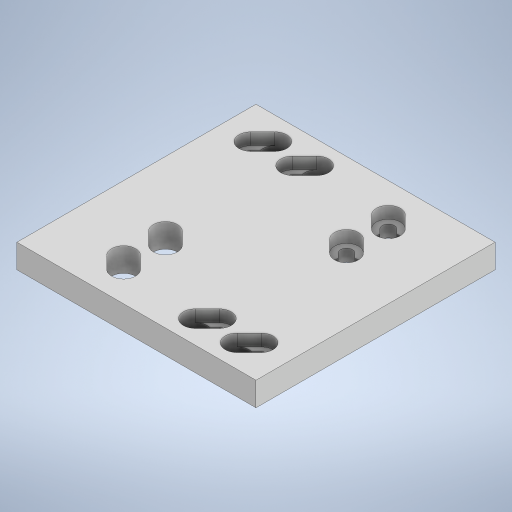
# Autodesk Inventor part: middle
Saved by Autodesk Inventor 2023 (Build 270158000, 158)
## iProperties
Created: 2023-08-09
Part Number: middle
Material: Generic
Document SubType Name: Modeling
Designer: AxLab
Density: 1 g/cm^3
Appearance: Default
Author: AxLab
Autodesk Inventor part; units mm, degrees
ref_plane "YZ Plane" through (0, 0, 0) normal (1, 0, 0) x (0, 1, 0)
ref_plane "XZ Plane" through (0, 0, 0) normal (0, 1, 0) x (-1, 0, 0)
ref_plane "XY Plane" through (0, 0, 0) normal (0, 0, 1) x (1, 0, 0)
sketch "Sketch6" plane through (0, 0, 0) normal (0, 1, 0) x (-1, 0, 0)
  line L0 (20, 20) -> (-20, 20)
  line L1 (-20, 20) -> (-20, -20)
  line L2 (-20, -20) -> (20, -20)
  line L3 (20, -20) -> (20, 20)
  line L4 (20, 20) -> (-20, -20) construction
  line L5 (-20, 20) -> (20, -20) construction
  line L6 (2.15, 11.15) -> (-2.15, 11.15)
  line L7 (-2.15, 11.15) -> (-2.15, -11.15)
  line L8 (-2.15, -11.15) -> (2.15, -11.15)
  line L9 (2.15, -11.15) -> (2.15, 11.15)
  line L10 (2.15, 11.15) -> (-2.15, -11.15) construction
  line L11 (-2.15, 11.15) -> (2.15, -11.15) construction
  line L12 (2.15, -11.15) -> (-20, -11.15)
  line L13 (-20, -11.15) -> (-20, -20)
  line L14 (-20, -20) -> (2.15, -20)
  line L15 (2.15, -20) -> (2.15, -11.15)
  line L16 (-2.15, 11.15) -> (20, 11.15)
  line L17 (20, 11.15) -> (20, 20)
  line L18 (20, 20) -> (-2.15, 20)
  line L19 (-2.15, 20) -> (-2.15, 11.15)
  line L20 (-20, -11.15) -> (-15, -11.15)
  line L21 (-15, -11.15) -> (-15, -14.15)
  line L22 (-15, -14.15) -> (-20, -14.15)
  line L23 (-20, -14.15) -> (-20, -11.15)
  line L24 (-20, -11.15) -> (-8, -11.15)
  line L25 (-8, -11.15) -> (-8, -14.15)
  line L26 (-8, -14.15) -> (-20, -14.15)
  line L27 (-20, -14.15) -> (-20, -11.15)
  line L28 (-2.15, 20) -> (-7.15, 20)
  line L29 (-7.15, 20) -> (-7.15, 15)
  line L30 (-7.15, 15) -> (-2.15, 15)
  line L31 (-2.15, 15) -> (-2.15, 20)
  line L32 (-2.15, 20) -> (-7.15, 20)
  line L33 (-7.15, 20) -> (-7.15, 8)
  line L34 (-7.15, 8) -> (-2.15, 8)
  line L35 (-2.15, 8) -> (-2.15, 20)
  line L36 (20, 11.15) -> (15, 11.15)
  line L37 (15, 11.15) -> (15, 14.15)
  line L38 (15, 14.15) -> (20, 14.15)
  line L39 (20, 14.15) -> (20, 11.15)
  line L40 (20, 11.15) -> (8, 11.15)
  line L41 (8, 11.15) -> (8, 14.15)
  line L42 (8, 14.15) -> (20, 14.15)
  line L43 (20, 14.15) -> (20, 11.15)
  line L44 (2.15, -20) -> (7.15, -20)
  line L45 (7.15, -20) -> (7.15, -15)
  line L46 (7.15, -15) -> (2.15, -15)
  line L47 (2.15, -15) -> (2.15, -20)
  line L48 (2.15, -20) -> (7.15, -20)
  line L49 (7.15, -20) -> (7.15, -8)
  line L50 (7.15, -8) -> (2.15, -8)
  line L51 (2.15, -8) -> (2.15, -20)
  circle A0 centre (-13, -16.15) radius 2
  circle A1 centre (-6, -16.15) radius 2
  circle A2 centre (9.15, -13) radius 2
  circle A3 centre (9.15, -6) radius 2
  circle A4 centre (6, 16.15) radius 2
  circle A5 centre (13, 16.15) radius 2
  circle A6 centre (-9.15, 6) radius 2
  circle A7 centre (-9.15, 13) radius 2
  line L52 (-13, -16.15) -> (-15, -16.15)
  line L53 (-15, -16.15) -> (-15, -14.15)
  line L54 (-15, -14.15) -> (-13, -14.15)
  line L55 (-13, -14.15) -> (-13, -16.15)
  line L56 (-6, -16.15) -> (-8, -16.15)
  line L57 (-8, -16.15) -> (-8, -14.15)
  line L58 (-8, -14.15) -> (-6, -14.15)
  line L59 (-6, -14.15) -> (-6, -16.15)
  line L60 (9.15, -13) -> (7.15, -13)
  line L61 (7.15, -13) -> (7.15, -15)
  line L62 (7.15, -15) -> (9.15, -15)
  line L63 (9.15, -15) -> (9.15, -13)
  line L64 (9.15, -6) -> (7.15, -6)
  line L65 (7.15, -6) -> (7.15, -8)
  line L66 (7.15, -8) -> (9.15, -8)
  line L67 (9.15, -8) -> (9.15, -6)
  line L68 (13, 16.15) -> (15, 16.15)
  line L69 (15, 16.15) -> (15, 14.15)
  line L70 (15, 14.15) -> (13, 14.15)
  line L71 (13, 14.15) -> (13, 16.15)
  line L72 (6, 16.15) -> (8, 16.15)
  line L73 (8, 16.15) -> (8, 14.15)
  line L74 (8, 14.15) -> (6, 14.15)
  line L75 (6, 14.15) -> (6, 16.15)
  line L76 (-9.15, 13) -> (-7.15, 13)
  line L77 (-7.15, 13) -> (-7.15, 15)
  line L78 (-7.15, 15) -> (-9.15, 15)
  line L79 (-9.15, 15) -> (-9.15, 13)
  line L80 (-9.15, 6) -> (-7.15, 6)
  line L81 (-7.15, 6) -> (-7.15, 8)
  line L82 (-7.15, 8) -> (-9.15, 8)
  line L83 (-9.15, 8) -> (-9.15, 6)
  line L84 (-15, -14.15) -> (-13, -16.15) construction
  line L85 (-16.4142, -15.5642) -> (-14.4142, -17.5642)
  line L86 (-11.5858, -14.7358) -> (-13.5858, -12.7358)
  arc A8 (-13.5858, -12.7358) -> (-16.4142, -15.5642) centre (-15, -14.15) ccw
  arc A9 (-14.4142, -17.5642) -> (-11.5858, -14.7358) centre (-13, -16.15) ccw
  line L87 (-8, -14.15) -> (-6, -16.15) construction
  line L88 (-9.4142, -15.5642) -> (-7.4142, -17.5642)
  line L89 (-4.5858, -14.7358) -> (-6.5858, -12.7358)
  arc A10 (-6.5858, -12.7358) -> (-9.4142, -15.5642) centre (-8, -14.15) ccw
  arc A11 (-7.4142, -17.5642) -> (-4.5858, -14.7358) centre (-6, -16.15) ccw
  line L90 (7.15, -15) -> (9.15, -13) construction
  line L91 (8.5642, -16.4142) -> (10.5642, -14.4142)
  line L92 (7.7358, -11.5858) -> (5.7358, -13.5858)
  arc A12 (5.7358, -13.5858) -> (8.5642, -16.4142) centre (7.15, -15) ccw
  arc A13 (10.5642, -14.4142) -> (7.7358, -11.5858) centre (9.15, -13) ccw
  line L93 (7.15, -8) -> (9.15, -6) construction
  line L94 (8.5642, -9.4142) -> (10.5642, -7.4142)
  line L95 (7.7358, -4.5858) -> (5.7358, -6.5858)
  arc A14 (5.7358, -6.5858) -> (8.5642, -9.4142) centre (7.15, -8) ccw
  arc A15 (10.5642, -7.4142) -> (7.7358, -4.5858) centre (9.15, -6) ccw
  line L96 (15, 14.15) -> (13, 16.15) construction
  line L97 (16.4142, 15.5642) -> (14.4142, 17.5642)
  line L98 (11.5858, 14.7358) -> (13.5858, 12.7358)
  arc A16 (13.5858, 12.7358) -> (16.4142, 15.5642) centre (15, 14.15) ccw
  arc A17 (14.4142, 17.5642) -> (11.5858, 14.7358) centre (13, 16.15) ccw
  line L99 (8, 14.15) -> (6, 16.15) construction
  line L100 (9.4142, 15.5642) -> (7.4142, 17.5642)
  line L101 (4.5858, 14.7358) -> (6.5858, 12.7358)
  arc A18 (6.5858, 12.7358) -> (9.4142, 15.5642) centre (8, 14.15) ccw
  arc A19 (7.4142, 17.5642) -> (4.5858, 14.7358) centre (6, 16.15) ccw
  line L102 (-7.15, 15) -> (-9.15, 13) construction
  line L103 (-8.5642, 16.4142) -> (-10.5642, 14.4142)
  line L104 (-7.7358, 11.5858) -> (-5.7358, 13.5858)
  arc A20 (-5.7358, 13.5858) -> (-8.5642, 16.4142) centre (-7.15, 15) ccw
  arc A21 (-10.5642, 14.4142) -> (-7.7358, 11.5858) centre (-9.15, 13) ccw
  line L105 (-7.15, 8) -> (-9.15, 6) construction
  line L106 (-8.5642, 9.4142) -> (-10.5642, 7.4142)
  line L107 (-7.7358, 4.5858) -> (-5.7358, 6.5858)
  arc A22 (-5.7358, 6.5858) -> (-8.5642, 9.4142) centre (-7.15, 8) ccw
  arc A23 (-10.5642, 7.4142) -> (-7.7358, 4.5858) centre (-9.15, 6) ccw
  line L108 (9.15, -13) -> (7.15, -15) construction
  line L109 (8.4429, -12.2929) -> (6.4429, -14.2929)
  line L110 (7.8571, -15.7071) -> (9.8571, -13.7071)
  arc A24 (9.8571, -13.7071) -> (8.4429, -12.2929) centre (9.15, -13) ccw
  arc A25 (6.4429, -14.2929) -> (7.8571, -15.7071) centre (7.15, -15) ccw
  line L111 (-6, -16.15) -> (-8, -14.15) construction
  line L112 (-5.2929, -15.4429) -> (-7.2929, -13.4429)
  line L113 (-8.7071, -14.8571) -> (-6.7071, -16.8571)
  arc A26 (-6.7071, -16.8571) -> (-5.2929, -15.4429) centre (-6, -16.15) ccw
  arc A27 (-7.2929, -13.4429) -> (-8.7071, -14.8571) centre (-8, -14.15) ccw
  line L114 (-13, -16.15) -> (-15, -14.15) construction
  line L115 (-12.2929, -15.4429) -> (-14.2929, -13.4429)
  line L116 (-15.7071, -14.8571) -> (-13.7071, -16.8571)
  arc A28 (-13.7071, -16.8571) -> (-12.2929, -15.4429) centre (-13, -16.15) ccw
  arc A29 (-14.2929, -13.4429) -> (-15.7071, -14.8571) centre (-15, -14.15) ccw
  line L117 (9.15, -6) -> (7.15, -8) construction
  line L118 (8.4429, -5.2929) -> (6.4429, -7.2929)
  line L119 (7.8571, -8.7071) -> (9.8571, -6.7071)
  arc A30 (9.8571, -6.7071) -> (8.4429, -5.2929) centre (9.15, -6) ccw
  arc A31 (6.4429, -7.2929) -> (7.8571, -8.7071) centre (7.15, -8) ccw
  line L120 (15, 14.15) -> (13, 16.15) construction
  line L121 (15.7071, 14.8571) -> (13.7071, 16.8571)
  line L122 (12.2929, 15.4429) -> (14.2929, 13.4429)
  arc A32 (14.2929, 13.4429) -> (15.7071, 14.8571) centre (15, 14.15) ccw
  arc A33 (13.7071, 16.8571) -> (12.2929, 15.4429) centre (13, 16.15) ccw
  line L123 (6, 16.15) -> (8, 14.15) construction
  line L124 (5.2929, 15.4429) -> (7.2929, 13.4429)
  line L125 (8.7071, 14.8571) -> (6.7071, 16.8571)
  arc A34 (6.7071, 16.8571) -> (5.2929, 15.4429) centre (6, 16.15) ccw
  arc A35 (7.2929, 13.4429) -> (8.7071, 14.8571) centre (8, 14.15) ccw
  line L126 (-7.15, 8) -> (-9.15, 6) construction
  line L127 (-7.8571, 8.7071) -> (-9.8571, 6.7071)
  line L128 (-8.4429, 5.2929) -> (-6.4429, 7.2929)
  arc A36 (-6.4429, 7.2929) -> (-7.8571, 8.7071) centre (-7.15, 8) ccw
  arc A37 (-9.8571, 6.7071) -> (-8.4429, 5.2929) centre (-9.15, 6) ccw
  line L129 (-7.15, 15) -> (-9.15, 13) construction
  line L130 (-7.8571, 15.7071) -> (-9.8571, 13.7071)
  line L131 (-8.4429, 12.2929) -> (-6.4429, 14.2929)
  arc A38 (-6.4429, 14.2929) -> (-7.8571, 15.7071) centre (-7.15, 15) ccw
  arc A39 (-9.8571, 13.7071) -> (-8.4429, 12.2929) centre (-9.15, 13) ccw
  point P0 (0, 0)
  point P1 (-14, -15.15)
  point P2 (-7, -15.15)
  point P3 (8.15, -14)
  point P4 (8.15, -7)
  point P5 (14, 15.15)
  point P6 (7, 15.15)
  point P7 (-8.15, 14)
  point P8 (-8.15, 7)
  point P9 (8.15, -14)
  point P10 (-7, -15.15)
  point P11 (-14, -15.15)
  point P12 (8.15, -7)
  point P13 (14, 15.15)
  point P14 (7, 15.15)
  point P15 (-8.15, 7)
  point P16 (-8.15, 14)
  dimension "d79" = 40
  dimension "d80" = 40
  dimension "d81" = 4.3
  dimension "d82" = 22.3
  dimension "d83" = 5
  dimension "d84" = 3
  dimension "d85" = 12
  dimension "d86" = 5
  dimension "d87" = 5
  dimension "d88" = 12
  dimension "d93" = 5
  dimension "d94" = 3
  dimension "d95" = 12
  dimension "d96" = 5
  dimension "d97" = 5
  dimension "d98" = 12
  dimension "d127" = 4
  dimension "d128" = 4
  dimension "d129" = 4
  dimension "d130" = 4
  dimension "d131" = 4
  dimension "d132" = 4
  dimension "d133" = 4
  dimension "d134" = 4
  dimension "d137" = 4
  dimension "d140" = 2
  dimension "d141" = 2
  dimension "d142" = 2
  dimension "d143" = 2
  dimension "d144" = 2
  dimension "d145" = 2
  dimension "d146" = 2
  dimension "d147" = 2
  constraints: 296 end point, 65 equal length, 64 point on circle, 64 tangent, 40 centre point, 24 perpendicular, 20 horizontal, 20 midpoint, 8 concentric, 4 point on line
  measures "d79" distance of L2.end L1.end
  measures "d80" distance of L1.end L0.end
  measures "d81" distance of L8.end L7.end
  measures "d82" distance of L7.end L6.end
  measures "d83" distance of L21.end L22.end
  measures "d84" distance of L20.end L21.end
  measures "d85" distance of L25.end L26.end
  measures "d86" distance of L30.end L29.end
  measures "d87" distance of L29.end L28.end
  measures "d88" distance of L33.end L32.end
  measures "d93" distance of L37.end L38.end
  measures "d94" distance of L36.end L37.end
  measures "d95" distance of L41.end L42.end
  measures "d96" distance of L46.end L45.end
  measures "d97" distance of L45.end L44.end
  measures "d98" distance of L49.end L48.end
  measures "d127" diameter of A0
  measures "d128" diameter of A1
  measures "d129" diameter of A2
  measures "d130" diameter of A3
  measures "d131" diameter of A4
  measures "d132" diameter of A5
  measures "d133" diameter of A6
  measures "d134" diameter of A7
  measures "d137" diameter of A9
  measures "d140" diameter of A25
  measures "d141" diameter of A27
  measures "d142" diameter of A29
  measures "d143" diameter of A31
  measures "d144" diameter of A33
  measures "d145" diameter of A35
  measures "d146" diameter of A37
  measures "d147" diameter of A39
extrude "Extrusion9" add sketch "Sketch6" along normal blind 4 contours L3 L38 A16 L97 A5 L98 L42 A18 L100 A4 L101 L41 L16 L6 L19 L0 | L19 L30 A20 L29 L0 | L3 L16 L37 A16 L38 | L29 A20 L103 A7 L104 L33 A22 L106 A6 L107 L34 L7 L12 L1 L0 | L19 L7 L34 A22 L33 L104 A20 L30 | L3 L2 L45 A12 L91 A2 L92 L49 A14 L94 A3 L95 L50 L9 L16 | A16 L37 A32 L38 | L38 A32 L121 L69 A5 L97 A16 | A20 L30 A38 L29 | L29 A38 L130 L78 A7 L103 A20 | L6 L9 L8 L7 | A20 L104 L33 L131 A38 L30 | L16 L41 A18 L42 L98 A16 L37 | A32 L37 L38 | L38 L69 L121 A32 | A16 L98 L42 L122 A32 L37 | L12 L21 A8 L22 L1 | A38 L30 L29 | L29 L78 L130 A38 | A38 L131 L33 L30 | L2 L15 L46 A12 L45 | L37 A32 L122 L42 | L42 L122 A5 L121 L69 | L22 A8 L85 A0 L86 L26 A10 L88 A1 L89 L25 L12 L8 L15 L2 L1 | L12 L25 A10 L26 L86 A8 L21 | L33 L131 A7 L130 L78 | L50 A14 L49 L92 A12 L46 L15 L9 | A22 L107 A6 L81 L128 A36 L34 | L34 A36 L33 A22 | L104 A7 L33 | A12 L46 A25 L45 | L45 A25 L110 L62 A2 L91 A12 | A18 L101 A4 L74 L124 A35 L41 | L41 A35 L42 A18 | L42 A5 L122 | L121 A5 L69 | L98 A5 L42 | A8 L21 A29 L22 | L22 A29 L116 L53 A0 L85 A8 | A8 L86 L26 L115 A29 L21 | L33 A7 L131 | L130 A7 L78 | A14 L95 A3 L65 L118 A31 L50 | L50 A31 L49 A14 | A36 L128 L81 L34 | L34 L33 A36 | L33 A36 L127 L82 A6 L106 A22 | A25 L46 L45 | L45 L62 L110 A25 | A12 L92 L49 L109 A25 L46 | A35 L124 L74 L41 | L41 L42 A35 | L42 A35 L125 L73 A4 L100 A18 | A29 L21 L22 | L22 L53 L116 A29 | A10 L89 A1 L58 L112 A27 L25 | L25 A27 L26 A10 | A29 L115 L26 L21 | A31 L118 L65 L50 | L50 L49 A31 | L49 A31 L119 L66 A3 L94 A14 | L82 L127 A36 L33 | L81 L128 A6 L127 L82 | L46 A25 L109 L49 | L49 L109 A2 L110 L62 | L73 L125 A35 L42 | L74 L124 A4 L125 L73 | L26 L115 A0 L116 L53 | A27 L112 L58 L25 | L25 L26 A27 | L26 A27 L113 L57 A1 L88 A10 | L86 A0 L26 | L66 L119 A31 L49 | L65 L118 A3 L119 L66 | L92 A2 L49 | L81 A6 L128 | L127 A6 L82 | L49 A2 L109 | L110 A2 L62 | L125 A4 L73 | L74 A4 L124 | L26 A0 L115 | L116 A0 L53 | L57 L113 A27 L26 | L58 L112 A1 L113 L57 | L65 A3 L118 | L119 A3 L66 | L113 A1 L57 | L58 A1 L112
extrude "Extrusion10" cut sketch "Sketch6" along normal blind 2 contours A16 L37 A32 L38 | L38 A32 L121 L69 A5 L97 A16 | A20 L30 A38 L29 | L29 A38 L130 L78 A7 L103 A20 | A20 L104 L33 L131 A38 L30 | A32 L37 L38 | L38 L69 L121 A32 | A16 L98 L42 L122 A32 L37 | A38 L30 L29 | L29 L78 L130 A38 | A38 L131 L33 L30 | L37 A32 L122 L42 | L42 L122 A5 L121 L69 | A5 L68 L121 A33 L122 L71 | L33 L131 A7 L130 L78 | A7 L79 L130 A39 L131 L76 | A22 L107 A6 L81 L128 A36 L34 | L34 A36 L33 A22 | L104 A7 L33 | A12 L46 A25 L45 | L45 A25 L110 L62 A2 L91 A12 | A18 L101 A4 L74 L124 A35 L41 | L41 A35 L42 A18 | L42 A5 L122 | L121 A5 L69 | L98 A5 L42 | A5 L121 L68 | A8 L21 A29 L22 | L22 A29 L116 L53 A0 L85 A8 | A8 L86 L26 L115 A29 L21 | L33 A7 L131 | L130 A7 L78 | A7 L130 L79 | A14 L95 A3 L65 L118 A31 L50 | L50 A31 L49 A14 | A36 L128 L81 L34 | L34 L33 A36 | L33 A36 L127 L82 A6 L106 A22 | L76 L131 A7 | A25 L46 L45 | L45 L62 L110 A25 | A12 L92 L49 L109 A25 L46 | A35 L124 L74 L41 | L41 L42 A35 | L42 A35 L125 L73 A4 L100 A18 | L71 L122 A5 | L122 L71 L68 L121 A5 | L68 L71 L122 A33 L121 | A29 L21 L22 | L22 L53 L116 A29 | A10 L89 A1 L58 L112 A27 L25 | L25 A27 L26 A10 | A29 L115 L26 L21 | L131 L76 L79 L130 A7 | L79 L76 L131 A39 L130 | A31 L118 L65 L50 | L50 L49 A31 | L49 A31 L119 L66 A3 L94 A14 | L82 L127 A36 L33 | L81 L128 A6 L127 L82 | A6 L83 L127 A37 L128 L80 | L46 A25 L109 L49 | L49 L109 A2 L110 L62 | A2 L63 L110 A24 L109 L60 | L73 L125 A35 L42 | L74 L124 A4 L125 L73 | A4 L72 L125 A34 L124 L75 | L26 L115 A0 L116 L53 | A0 L52 L116 A28 L115 L55 | A27 L112 L58 L25 | L25 L26 A27 | L26 A27 L113 L57 A1 L88 A10 | L86 A0 L26 | L66 L119 A31 L49 | L65 L118 A3 L119 L66 | A3 L67 L119 A30 L118 L64 | L92 A2 L49 | L81 A6 L128 | L127 A6 L82 | L80 L128 A6 | L49 A2 L109 | L110 A2 L62 | A2 L110 L63 | L125 A4 L73 | L74 A4 L124 | L75 L124 A4 | L26 A0 L115 | L116 A0 L53 | A0 L116 L52 | L57 L113 A27 L26 | L58 L112 A1 L113 L57 | A1 L56 L113 A26 L112 L59 | L55 L115 A0 | L65 A3 L118 | L119 A3 L66 | L64 L118 A3 | L60 L109 A2 | L128 L80 L83 L127 A6 | A6 L127 L83 | L128 A37 L127 L83 L80 | L109 L60 L63 L110 A2 | L63 L60 L109 A24 L110 | A4 L125 L72 | A4 L124 L75 L72 L125 | L124 A34 L125 L72 L75 | L115 L55 L52 L116 A0 | L52 L55 L115 A28 L116 | L113 A1 L57 | L58 A1 L112 | L59 L112 A1 | L118 L64 L67 L119 A3 | A3 L119 L67 | L118 A30 L119 L67 L64 | A1 L113 L56 | A1 L112 L59 L56 L113 | L112 A26 L113 L56 L59
extrude "Extrusion11" cut sketch "Sketch6" along normal blind 4 contours A32 L37 L38 | L38 L69 L121 A32 | A38 L30 L29 | L29 L78 L130 A38 | A38 L131 L33 L30 | L37 A32 L122 L42 | L42 L122 A5 L121 L69 | L33 L131 A7 L130 L78 | A36 L128 L81 L34 | L34 L33 A36 | A25 L46 L45 | L45 L62 L110 A25 | A35 L124 L74 L41 | L41 L42 A35 | L122 L71 L68 L121 A5 | L68 L71 L122 A33 L121 | A29 L21 L22 | L22 L53 L116 A29 | A29 L115 L26 L21 | L131 L76 L79 L130 A7 | L79 L76 L131 A39 L130 | A31 L118 L65 L50 | L50 L49 A31 | L82 L127 A36 L33 | L81 L128 A6 L127 L82 | L46 A25 L109 L49 | L49 L109 A2 L110 L62 | L73 L125 A35 L42 | L74 L124 A4 L125 L73 | L26 L115 A0 L116 L53 | A27 L112 L58 L25 | L25 L26 A27 | L66 L119 A31 L49 | L65 L118 A3 L119 L66 | L57 L113 A27 L26 | L58 L112 A1 L113 L57 | L128 L80 L83 L127 A6 | L128 A37 L127 L83 L80 | L109 L60 L63 L110 A2 | L63 L60 L109 A24 L110 | A4 L124 L75 L72 L125 | L124 A34 L125 L72 L75 | L115 L55 L52 L116 A0 | L52 L55 L115 A28 L116 | L118 L64 L67 L119 A3 | L118 A30 L119 L67 L64 | A1 L112 L59 L56 L113 | L112 A26 L113 L56 L59
move or copy body "Move Body1" bodies to move or copy 1 copy no rotation origin (0, 0, 0) rotation axis (0, 0, 1) rotation angle 180
body "Solid4"
